screw_wheel_60_m3 (Autodesk Fusion 360 design; units mm, degrees)
Autodesk Fusion 360 part; units mm, degrees
sketch "Sketch1" plane through (0, 0, 0) normal (0, 1, 0) x (1, 0, 0)
  circle A0 centre (0, 0) radius 27.5
  circle A1 centre (0, 0) radius 1.6
  dimension "d1" = 55
  dimension "d2" = 3.2
  constraint coincident A0.centre A1.centre
  constraint concentric A0 A1
  measures "d1" diameter of A0
  measures "d2" diameter of A1
extrude "Extrude1" add sketch "Sketch1" along normal blind 4 contours A0 picked at (18.764283, -1.366221)
fillet "Fillet1" radius 1 2 edges at (-25.639002, 0, 9.944424) (-25.639002, 4, 9.944424)
sketch "Sketch2" plane through (0, 0, 0) normal (0, -1, 0) x (1, 0, 0)
  circle A0 centre (0, 0) radius 1.6
  circle A1 centre (0, 0) radius 26.5
  circle A2 centre (0, 0) radius 27.5
  circle A3 centre (0, 27.5) radius 0.75
  circle A4 centre (-1.195778, 26.873409) radius 0.6
  circle A5 centre (1.195778, 26.873409) radius 0.6
  dimension "d7" = 1.5
  dimension "d8" = 1.2
  constraint coincident A2 A3.centre
  constraint vertical A0.centre A3.centre
  constraint tangent A2 A4
  constraint tangent A3 A4
  constraint tangent A3 A5
  constraint tangent A2 A5
  constraint equal A4 A5
  measures "d7" diameter of A3
  measures "d8" diameter of A4
extrude "Extrude2" cut sketch "Sketch2" against normal through all contours A2 A3 A4 | A2 A3 | A2 A3 A5 picked at (-0.851365, 27.456117) picked at (0.01812, 27.2499) picked at (0.851365, 27.456117)
pattern_circular "C-Pattern1" count 62 over 360 about axis through (0, 1.75, 0) along (0, 1, 0) of "Extrude2"
sketch "Sketch3" plane through (0, 0, 0) normal (0, -1, 0) x (1, 0, 0)
  circle A0 centre (0, 0) radius 1.6
  circle A1 centre (0, 0) radius 26.5
  line L0 (-1.645448, 2.85) -> (-3.290897, 0)
  line L1 (-3.290897, 0) -> (-1.645448, -2.85)
  line L2 (-1.645448, -2.85) -> (1.645448, -2.85)
  line L3 (1.645448, -2.85) -> (3.290897, 0)
  line L4 (3.290897, 0) -> (1.645448, 2.85)
  line L5 (1.645448, 2.85) -> (-1.645448, 2.85)
  dimension "d12" = 5.7
  constraint coincident A0.centre A1.centre
  measures "d12" distance of L2 L5
extrude "Extrude3" cut sketch "Sketch3" against normal blind 3.5 contours L0 L1 L2 L3 L4 L5 picked at (-2.125965, 1.181405)
sketch "Sketch4" plane through (0, 0, 0) normal (0, -1, 0) x (1, 0, 0)
  line L0 (-3.290897, 0) -> (-1.645448, 2.85)
  line L1 (-1.645448, 2.85) -> (1.645448, 2.85)
  line L2 (1.645448, 2.85) -> (3.290897, 0)
  line L3 (3.290897, 0) -> (1.645448, -2.85)
  line L4 (1.645448, -2.85) -> (-1.645448, -2.85)
  line L5 (-1.645448, -2.85) -> (-3.290897, 0)
  circle A0 centre (0, 0) radius 26.5
  line L6 (0, 0) -> (-6.014116, 19.074339)
  line L7 (6.014116, 19.074339) -> (0, 0)
  line L8 (0, 0) -> (0, 20) construction
  arc A1 (6.014116, 19.074339) -> (-6.014116, 19.074339) centre (0, 0) ccw
  arc A2 (2.405646, 7.629736) -> (-2.405646, 7.629736) centre (0, 0) ccw
  arc A3 (-3.857506, 19.624466) -> (-5.379189, 17.060607) centre (-3.471755, 17.662019) ccw
  arc A4 (5.379189, 17.060607) -> (3.857506, 19.624466) centre (3.471755, 17.662019) ccw
  arc A5 (0.831095, 7.956713) -> (2.946303, 9.34448) centre (1.038869, 9.945891) ccw
  arc A6 (-2.946303, 9.34448) -> (-0.831095, 7.956713) centre (-1.038869, 9.945891) ccw
  dimension "d15" = 40
  dimension "d17" = 35
  dimension "d18" = 17.5
  dimension "d23" = 8
  dimension "d24" = 4
  constraint concentric A0 A1
  constraint coincident A0.centre L6.start
  constraint coincident L8.end A1
  constraint vertical L8
  constraint coincident A0.centre L8
  constraint equal A3 A4
  constraint equal A4 A5
  constraint equal A5 A6
  constraint tangent A1 A3
  constraint tangent L6 A3
  constraint tangent A1 A4
  constraint tangent L7 A4
  constraint tangent L7 A5
  constraint tangent A2 A5
  constraint tangent A2 A6
  constraint tangent L6 A6
  measures "d15" diameter of A1
  measures "d17" angle of L6 L7
  measures "d18" angle of L6 L8
  measures "d23" radius of A2
  measures "d24" diameter of A3
extrude "Extrude4" cut sketch "Sketch4" against normal through all contours L6 L7 A1 A2 A3 A4 A5 A6 picked at (0.431014, 12.882372)
pattern_circular "C-Pattern2" count 6 over 360 about axis through (0, 1.75, 0) along (0, 1, 0) of "Extrude4"
equation "d18 = d17 / 2"
